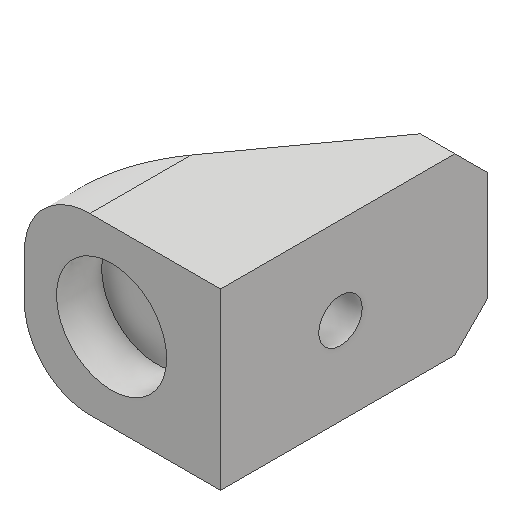
# Autodesk Inventor part: 3DP_ABS_Front_Door_Frame_Magnet_Mount
Saved by Autodesk Inventor 2026.1 (Build 301233000, 233)
## iProperties
Created: 2016-06-27
Part Number: 3DP_ABS_Front_Door_Frame_Magnet_Mount
Material: Ogólny
Document SubType Name: Modeling
Designer: Andrzej
Density: 1 g/cm^3
Appearance: Domyślna
Author: Andrzej
Autodesk Inventor part; units mm, degrees
ref_plane "YZ Plane" through (0, 0, 0) normal (1, 0, 0) x (0, 1, 0)
ref_plane "XZ Plane" through (0, 0, 0) normal (0, 1, 0) x (-1, 0, 0)
ref_plane "XY Plane" through (0, 0, 0) normal (0, 0, 1) x (1, 0, 0)
sketch "Szkic1" plane through (0, 0, 0) normal (0, 0, 1) x (1, 0, 0)
  line L0 (0, 0.1419) -> (0, -24.3581)
  line L1 (0, -24.3581) -> (-18, -24.3581)
  line L2 (-18, -24.3581) -> (-18, -23.3581)
  line L3 (0, 0.1419) -> (-1, 0.1419)
  line L4 (-1, 0.1419) -> (-18, -23.3581)
  point P0 (0, 0)
  dimension "d0" = 24.5
  dimension "d1" = 18
  dimension "d2" = 1
  dimension "d3" = 1
  constraints: 10 end point, 2 vertical, 1 horizontal, 1 perpendicular
  measures "d0" distance of L0.start L0.end
  measures "d1" distance of L0.end L1.end
  measures "d2" distance of L1.end L2.end
  measures "d3" distance of L0.start L3.end
extrude "Wyciągnięcie proste1" add sketch "Szkic1" along normal blind 16
sketch "Szkic2" plane through (0, -24.3581, 0) normal (1, 0, 0) x (0, 0, -1)
  line L0 (0, 24.5) -> (0, 0) projected
  line L1 (0, 24.5) -> (-16, 24.5) projected
  line L2 (-16, 0) -> (-16, 24.5) projected
  line L3 (0, 0) -> (-16, 0) projected
  point P0 (0, 24.3581)
  point P1 (-8, 11)
  dimension "d6" = 16
  dimension "d7" = 13.5
  dimension "d8" = 8
  measures "d6" distance of L0.start L1.end
  measures "d7" distance from line of L1 point (-8, 11)
  measures "d8" distance from line of L2 point (-8, 11)
hole "Otwór1" at (0, -13.3581, 8) direction (-1, 0, 0) diameter 4 end through all
sketch "Szkic3" plane through (-18, -24.3581, 0) normal (0, -1, 0) x (1, 0, 0)
  line L0 (18, 0) -> (0, 0) projected
  line L1 (18, 0) -> (18, 16) projected
  line L2 (0, 16) -> (18, 16) projected
  line L3 (0, 0) -> (0, 16) projected
  circle A0 centre (8, 8) radius 5.05
  dimension "d16" = 10.1
  dimension "d17" = 10
  dimension "d18" = 16
  dimension "d19" = 8
  constraints: 1 centre point
  measures "d16" diameter of A0
  measures "d17" distance from line of L1 A0.centre
  measures "d18" distance of L0.end L2.start
  measures "d19" distance from line of L2 A0.centre
extrude "Wyciągnięcie proste2" cut sketch "Szkic3" against normal blind 4.15 contours A0
sketch "Szkic4" plane through (-18, -24.3581, 0) normal (-1, 0, 0) x (0, 0, 1)
  circle A0 centre (8, 11) radius 2 projected
  circle A1 centre (8, 11) radius 4.5
  point P0 (0, 24.3581)
  dimension "d22" = 9
  constraints: 1 centre point, 1 coincident
  measures "d22" diameter of A1
extrude "Wyciągnięcie proste3" cut sketch "Szkic4" against normal blind 15
fillet "Zaokrąglenie1" radius 6 2 edges at (-18, -23.8581, 16) (-18, -23.8581, 0)
chamfer "Faza1" distance 3 angle 45 2 edges at (-0.5, 0.1419, 16) (-0.5, 0.1419, 0)
equation "\"d8\" = 0.5 * d6"
equation "\"d19\" = 0.5 * d18"
